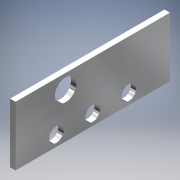
# Autodesk Inventor part: Inner Plate
Saved by Autodesk Inventor 2019.4 (Build 234330000, 330)
## iProperties
Created: 2019-12-07
Part Number: Inner Plate
Material: Aluminum 6061
Document SubType Name: Modeling
Designer: admin
Density: 2.7 g/cm^3
Appearance: Aluminum - Flat
Mass: 453.945 g
Surface Area: 568.361 cm^2
Volume: 168.128 cm^3
Author: admin
Autodesk Inventor part; units mm, degrees
ref_plane "YZ Plane" through (0, 0, 0) normal (1, 0, 0) x (0, 1, 0)
ref_plane "XZ Plane" through (0, 0, 0) normal (0, 1, 0) x (-1, 0, 0)
ref_plane "XY Plane" through (0, 0, 0) normal (0, 0, 1) x (1, 0, 0)
sketch "Sketch1" plane through (0, 0, 0) normal (1, 0, 0) x (0, 1, 0)
  line L0 (49.2406, -203.3994) -> (-27.7594, -203.3994)
  line L1 (-27.7594, -203.3994) -> (-27.7594, -3.3994)
  line L2 (-27.7594, -3.3994) -> (49.2406, -3.3994)
  line L3 (49.2406, -3.3994) -> (49.2406, -203.3994)
  line L4 (32.2406, -193.3994) -> (32.2406, -13.3994) construction
  line L5 (32.2406, -103.3994) -> (2.7957, -103.3994) construction
  point P0 (0, 0)
  dimension "d2" = 77
  dimension "d3" = 200
  dimension "d7" = 180
  dimension "d8" = 60
  dimension "d9" = 100
  constraints: 12 end point, 2 horizontal, 2 parallel, 1 midpoint, 1 perpendicular, 1 vertical
  measures "d2" distance of L0.start L0.end
  measures "d3" distance of L2.end L0.start
  measures "d7" distance of L4.end L4.start
  measures "d8" distance between parallel lines of L1 L4
  measures "d9" distance between parallel lines of L0 L5
extrude "Extrusion1" add sketch "Sketch1" along normal blind 7
sketch "Sketch2" plane through (7, 0, 0) normal (1, 0, 0) x (0, 0, -1)
  line L0 (203.3994, 49.2406) -> (3.3994, 49.2406) projected
  line L1 (103.3994, 49.2406) -> (103.3994, -27.7594) construction
  line L2 (3.3994, -27.7594) -> (203.3994, -27.7594) projected
  circle A0 centre (103.3994, -13.7594) radius 9.5
  circle A1 centre (56.4094, -13.7594) radius 9.5
  circle A2 centre (150.3894, -13.7594) radius 9.5
  circle A3 centre (68.3994, 30.2756) radius 14
  point P0 (0, 0)
  dimension "d10" = 19
  dimension "d11" = 63
  dimension "d14" = 19
  dimension "d15" = 19
  dimension "d16" = 63
  dimension "d17" = 63
  dimension "d18" = 46.99
  dimension "d19" = 46.99
  dimension "d22" = 28
  dimension "d23" = 18.965
  dimension "d24" = 11.99
  constraints: 4 centre point, 2 end point, 2 midpoint, 1 point on line
  measures "d10" diameter of A0
  measures "d11" distance from line of L0 A0.centre
  measures "d14" diameter of A1
  measures "d15" diameter of A2
  measures "d16" distance from line of L0 A2.centre
  measures "d17" distance from line of L0 A1.centre
  measures "d18" distance of A0.centre A1.centre
  measures "d19" distance of A0.centre A2.centre
  measures "d22" diameter of A3
  measures "d23" distance from line of L0 A3.centre
  measures "d24" horizontal distance of A1.centre A3.centre
extrude "Extrusion2" cut sketch "Sketch2" against normal blind 10
sketch "Sketch3" plane through (7, 0, 0) normal (1, 0, 0) x (0, 0, -1)
  line L0 (203.3994, 49.2406) -> (3.3994, 49.2406) projected
  line L1 (203.3994, 49.2406) -> (703.3994, 49.2406)
  line L2 (703.3994, 49.2406) -> (703.3994, -27.7594)
  line L3 (703.3994, -27.7594) -> (203.3994, -27.7594)
  line L4 (203.3994, -27.7594) -> (203.3994, 49.2406)
  point P0 (0, 0)
  dimension "d25" = 500
  dimension "d26" = 77
  constraints: 8 end point, 2 parallel, 1 horizontal, 1 perpendicular
  measures "d25" distance of L2.end L3.end
  measures "d26" distance of L1.end L2.end
extrude "Extrusion3" add sketch "Sketch3" against normal blind 7
sketch "Sketch4" plane through (7, 0, 0) normal (1, 0, 0) x (0, 0, -1)
  circle A0 centre (638.3994, 30.2756) radius 14
  line L0 (3.3994, 49.2406) -> (703.3994, 49.2406) projected
  line L1 (703.3994, 49.2406) -> (703.3994, -27.7594) projected
  line L2 (3.3994, -27.7594) -> (703.3994, -27.7594) projected
  line L3 (353.3994, -27.7594) -> (353.3994, 49.2406) construction
  circle A1 centre (353.3994, 30.2756) radius 14
  point P0 (0, 0)
  dimension "d29" = 28
  dimension "d30" = 18.965
  dimension "d31" = 65
  dimension "d32" = 77
  dimension "d33" = 28
  dimension "d34" = 18.965
  constraints: 2 centre point, 2 end point, 2 midpoint, 1 point on line
  measures "d29" diameter of A0
  measures "d30" distance from line of L0 A0.centre
  measures "d31" distance from line of L1 A0.centre
  measures "d32" distance of L3.start L3.end
  measures "d33" diameter of A1
  measures "d34" distance from line of L0 A1.centre
extrude "Extrusion4" cut sketch "Sketch4" against normal blind 7
equation "\"d9\" = 0.5 * d3"
equation "\"d11\" = d17"
equation "\"d16\" = d17"
body "Solid1"
